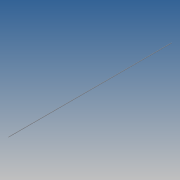
# Autodesk Inventor part: pipe1.5m
Saved by Autodesk Inventor 2014 SP1 (Build 180222100, 222)
## iProperties
Created: 2014-05-20
Part Number: pipe1.5m
Material: Generic
Document SubType Name: Modeling
Designer: Dave
Density: 1 g/cm^3
Appearance: Default
Author: Dave
Autodesk Inventor part; units mm, degrees
ref_plane "YZ Plane" through (0, 0, 0) normal (1, 0, 0) x (0, 1, 0)
ref_plane "XZ Plane" through (0, 0, 0) normal (0, 1, 0) x (-1, 0, 0)
ref_plane "XY Plane" through (0, 0, 0) normal (0, 0, 1) x (1, 0, 0)
sketch "Sketch1" plane through (0, 0, 0) normal (0, 0, 1) x (1, 0, 0)
  circle A0 centre (0, 0) radius 23.5
  circle A1 centre (0, 0) radius 26.5
  dimension "d0" = 47
  dimension "d1" = 3
  constraints: 2 centre point, 1 coincident
  measures "d0" diameter of A0
  measures "d1" radial gap between concentric circles of A1 A0
extrude "Extrusion1" add sketch "Sketch1" along normal blind 20000
body "Solid1"
